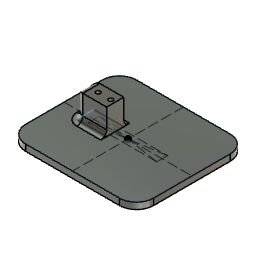
UF Plate v1.0 (Autodesk Fusion 360 design; units mm, degrees)
Autodesk Fusion 360 part; units mm, degrees
sketch "Sketch1" plane through (0, 0, 0) normal (0, 0, 1) x (1, 0, 0)
  line L0 (20, 0) -> (130, 0)
  line L1 (150, 20) -> (150, 110)
  line L2 (130, 130) -> (20, 130)
  line L3 (0, 110) -> (0, 20)
  arc A0 (20, 130) -> (0, 110) centre (20, 110) ccw
  arc A1 (150, 110) -> (130, 130) centre (130, 110) ccw
  arc A2 (130, 0) -> (150, 20) centre (130, 20) ccw
  arc A3 (0, 20) -> (20, 0) centre (20, 20) ccw
  point P0 (150, 0)
  point P1 (0, 130)
  dimension "d1" = 150
  dimension "d2" = 130
  dimension "d3" = 20
  constraint horizontal L0
  constraint vertical L1
  constraint horizontal L2
  constraint vertical L3
  constraint coincident P1 L2
  constraint coincident P1 L3
  constraint tangent L2 A0
  constraint tangent L3 A0
  constraint tangent L1 A1
  constraint tangent L2 A1
  constraint equal A0 A1
  constraint coincident P0 L0
  constraint coincident P0 L1
  constraint tangent L0 A2
  constraint tangent L1 A2
  constraint equal A0 A2
  constraint coincident origin L0
  constraint coincident origin L3
  constraint tangent L0 A3
  constraint tangent L3 A3
  constraint equal A0 A3
  measures "d1" distance of origin P0
  measures "d2" distance of origin P1
  measures "d3" radius of A0
extrude "Extrude1" add sketch "Sketch1" along normal blind 7.5
sketch "Sketch2" plane through (0, 0, 7.5) normal (0, 0, 1) x (-1, 0, 0)
  arc A0 (0, -20) -> (-20, 0) centre (-20, -20) ccw
  line L0 (-20, 0) -> (-130, 0)
  arc A1 (-130, 0) -> (-150, -20) centre (-130, -20) ccw
  line L1 (-150, -20) -> (-150, -110)
  arc A2 (-150, -110) -> (-130, -130) centre (-130, -110) ccw
  line L2 (-130, -130) -> (-20, -130)
  arc A3 (-20, -130) -> (0, -110) centre (-20, -110) ccw
  line L3 (0, -110) -> (0, -20)
  line L4 (-75, -130) -> (-75, 0) construction
  line L5 (0, -65) -> (-150, -65) construction
  line L6 (-115, -58.75) -> (-35, -58.75) construction
  line L7 (-35, -58.75) -> (-35, -71.25) construction
  line L8 (-35, -71.25) -> (-115, -71.25) construction
  line L9 (-115, -71.25) -> (-115, -58.75) construction
  line L10 (-115, -58.75) -> (-35, -71.25) construction
  line L11 (-35, -58.75) -> (-115, -71.25) construction
  line L12 (-35, -65) -> (-60, -65) construction
  line L13 (-60, -65) -> (-60, -75)
  line L14 (-60, -75) -> (-25, -75)
  line L15 (-60, -65) -> (-60, -55)
  line L16 (-60, -55) -> (-25, -55)
  line L17 (-25, -55) -> (-25, -75)
  point P0 (-75, -65)
  dimension "d6" = 80
  dimension "d7" = 12.5
  dimension "d10" = 25
  dimension "d11" = 10
  dimension "d12" = 10
  constraint midpoint L2 L4.start
  constraint midpoint L0 L4.end
  constraint midpoint L3 L5.start
  constraint midpoint L1 L5.end
  constraint horizontal L6
  constraint perpendicular L6 L7
  constraint parallel L6 L8
  constraint parallel L7 L9
  constraint coincident L10 P0
  constraint coincident L11 P0
  constraint midpoint L5 P0
  constraint midpoint L7 L12.start
  constraint perpendicular L7 L12
  constraint perpendicular L8 L13
  constraint perpendicular L13 L14
  constraint perpendicular L12 L15
  constraint perpendicular L4 L16
  constraint perpendicular L14 L17
  measures "d6" distance of L7.end L8.end
  measures "d7" distance of L6.end L7.end
  measures "d10" distance of L12.start L12.end
  measures "d11" distance of L12.end L13.end
  measures "d12" distance of L12.end L15.end
extrude "Extrude2" add sketch "Sketch2" along normal blind 30 contours L13 L14 L15 L16 L17
sketch "Sketch3" plane through (0, 0, 37.5) normal (0, 0, 1) x (-1, 0, 0)
  line L0 (-60, -55) -> (-60, -75)
  line L1 (-60, -75) -> (-25, -75)
  line L2 (-25, -75) -> (-25, -55)
  line L3 (-25, -55) -> (-60, -55)
  line L4 (-60, -65) -> (-35, -65) construction
  line L5 (-35, -65) -> (-40, -65) construction
  circle A0 centre (-40, -65) radius 2.5
  circle A1 centre (-55, -65) radius 2.5
  dimension "d15" = 5
  dimension "d18" = -15
  dimension "d19" = 0
  constraint midpoint L0 L4.start
  constraint perpendicular L0 L4
  constraint coincident L4 L5.end
  constraint coincident L5.end A0.centre
  measures "d15" diameter of A0
extrude "Extrude3" cut sketch "Sketch3" against normal blind 37.5 contours A0 | A1
sketch "Sketch4" plane through (0, 0, 0) normal (0, 0, -1) x (1, 0, 0)
  circle A0 centre (40, -65) radius 2.5
  circle A1 centre (55, -65) radius 2.5
  arc A2 (20, 0) -> (0, -20) centre (20, -20) ccw
  line L0 (0, -20) -> (0, -110)
  arc A3 (0, -110) -> (20, -130) centre (20, -110) ccw
  line L1 (20, -130) -> (130, -130)
  arc A4 (130, -130) -> (150, -110) centre (130, -110) ccw
  line L2 (150, -110) -> (150, -20)
  arc A5 (150, -20) -> (130, 0) centre (130, -20) ccw
  line L3 (130, 0) -> (20, 0)
  circle A6 centre (40, -65) radius 5
  circle A7 centre (55, -65) radius 5
  dimension "d22" = 10
  dimension "d23" = 10
  constraint concentric A0 A6
  constraint concentric A1 A7
  measures "d22" diameter of A6
  measures "d23" diameter of A7
extrude "Extrude4" cut sketch "Sketch4" against normal blind 7.5 contours A6 | A7
fillet "Fillet1" radius 7 6 edges at (25, 65, 7.5) (42.5, 55, 7.5) (25, 55, 22.5) (25, 75, 22.5) (25, 65, 37.5) (42.5, 75, 7.5)
